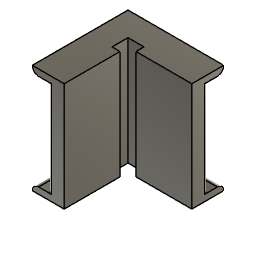
Tightening flaps (Autodesk Fusion 360 design; units mm, degrees)
Autodesk Fusion 360 part; units mm, degrees
sketch "Sketch1" plane through (0, 0, 0) normal (0, 0, 1) x (1, 0, 0)
  line L0 (50, 30) -> (110, 30)
  line L1 (110, 30) -> (110, 50)
  line L2 (110, 50) -> (50, 50)
  line L3 (50, 50) -> (50, 30)
  line L4 (110, 30) -> (60, 30)
  line L5 (60, 30) -> (60, 40)
  line L6 (60, 40) -> (110, 40)
  line L7 (110, 40) -> (110, 30)
  line L8 (50, 50) -> (70, 50)
  line L9 (70, 50) -> (70, -10)
  line L10 (70, -10) -> (50, -10)
  line L11 (50, -10) -> (50, 50)
  line L12 (60, 40) -> (70, 40)
  line L13 (70, 40) -> (70, -10)
  line L14 (70, -10) -> (60, -10)
  line L15 (60, -10) -> (60, 40)
  dimension "d1" = 60
  dimension "d2" = 20
  dimension "d3" = 50
  dimension "d4" = 10
  dimension "d5" = 20
  dimension "d6" = 60
  constraint horizontal L0
  constraint vertical L1
  constraint horizontal L2
  constraint vertical L3
  constraint horizontal L4
  constraint vertical L5
  constraint horizontal L6
  constraint vertical L7
  constraint horizontal L8
  constraint vertical L9
  constraint horizontal L10
  constraint vertical L11
  constraint horizontal L12
  constraint vertical L13
  constraint horizontal L14
  constraint vertical L15
  measures "d1" distance of L0.start L0.end
  measures "d2" distance of L0.start L2.end
  measures "d3" distance of L0.end L4.end
  measures "d4" distance of L0.end L6.end
  measures "d5" distance of L2.end L8.end
  measures "d6" distance of L2.end L10.end
extrude "Extrude1" add sketch "Sketch1" along normal blind 4 contours L0 L2 L3 L5 L6 L8 L9 L11 L12 L15 | L0 L10 L11 L15 | L1 L2 L6 L9
extrude "Extrude2" add sketch "Sketch1" along normal blind 64 contours L0 L4 L5 L6 L9 L12 L13 L15 | L0 L4 L9 L10 L13 L14 L15 | L0 L1 L4 L6 L7 L9 L13
sketch "Sketch2" plane through (0, 0, 64) normal (0, 0, 1) x (-1, 0, 0)
  line L0 (-60, 10) -> (-70, 10)
  line L1 (-70, 10) -> (-70, -30)
  line L2 (-70, -30) -> (-110, -30)
  line L3 (-110, -30) -> (-110, -40)
  line L4 (-110, -40) -> (-60, -40)
  line L5 (-60, -40) -> (-60, 10)
  line L6 (-70, 10) -> (-50, 10)
  line L7 (-50, 10) -> (-50, -50)
  line L8 (-50, -50) -> (-70, -50)
  line L9 (-70, -50) -> (-70, 10)
  line L10 (-70, -30) -> (-110, -30)
  line L11 (-110, -30) -> (-110, -50)
  line L12 (-110, -50) -> (-70, -50)
  line L13 (-70, -50) -> (-70, -30)
  constraint horizontal L6
  constraint vertical L7
  constraint horizontal L8
  constraint vertical L9
  constraint coincident L0.end L1.start
  constraint horizontal L10
  constraint vertical L11
  constraint horizontal L12
  constraint vertical L13
  constraint coincident L1.end L2.start
extrude "Extrude3" add sketch "Sketch2" along normal blind 4
sketch "Sketch3" plane through (0, 0, 68) normal (0, 0, 1) x (-1, 0, 0)
  line L0 (-70, -30) -> (-110, -30)
  line L1 (-110, -30) -> (-110, -50)
  line L2 (-110, -50) -> (-50, -50)
  line L3 (-50, -50) -> (-50, 10)
  line L4 (-50, 10) -> (-70, 10)
  line L5 (-70, 10) -> (-70, -30)
  line L6 (-75, -25) -> (-65, -25)
  line L7 (-65, -25) -> (-65, -35)
  line L8 (-65, -35) -> (-75, -35)
  line L9 (-75, -35) -> (-75, -25)
  constraint horizontal L6
  constraint vertical L7
  constraint horizontal L8
  constraint vertical L9
extrude "Extrude4" cut sketch "Sketch3" against normal blind 68 contours L0 L5 L6 L7 L8 L9
fillet "Fillet1" radius 4 2 edges at (80, 50, 4) (50, 20, 4)
fillet "Fillet2" radius 4 2 edges at (80, 50, 64) (50, 20, 64)
fillet "Fillet3" radius 2 1 edges at (110, 40, 34)
fillet "Fillet4" radius 2 1 edges at (60, -10, 34)
fillet "Fillet5" radius 2 1 edges at (60, 40, 34)
